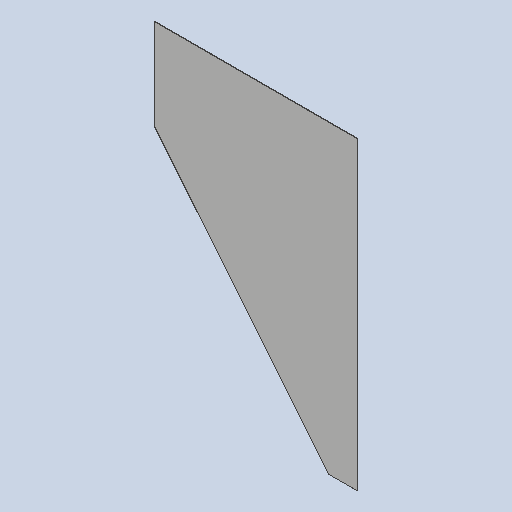
# Autodesk Inventor part: МОО 053 морда 3
Saved by Autodesk Inventor 2024.2 (Build 282272000, 272)
## iProperties
Created: 2024-06-08
Part Number: МОО 053 морда 3
Material: Generic
Document SubType Name: Sheet Metal
Designer: admin
Density: 1 g/cm^3
Sheet Metal Rule: Default
Appearance: Default
Author: admin
Autodesk Inventor part; units mm, degrees
ref_plane "YZ Plane" through (0, 0, 0) normal (1, 0, 0) x (0, 1, 0)
ref_plane "XZ Plane" through (0, 0, 0) normal (0, 1, 0) x (-1, 0, 0)
ref_plane "XY Plane" through (0, 0, 0) normal (0, 0, 1) x (1, 0, 0)
sketch "Sketch1" plane through (0, 0, 0) normal (0, 1, 0) x (-1, 0, 0)
  line L0 (0, 1200) -> (0, 0)
  line L1 (800, 843.901) -> (800, 1200)
  line L2 (800, 1200) -> (0, 1200)
  line L3 (800, 843.901) -> (113, 0)
  line L4 (113, 0) -> (0, 0)
  line L5 (685.2711, 713.7323) -> (114.1118, 12.1284)
  dimension "d0" = 1200
  dimension "d1" = 800
  dimension "d2" = 356.099
  dimension "d5" = 129.148
  dimension "d6" = 113
  measures "d0" distance of L0.end L0.start
  measures "d1" distance of L1.end L0.start
  measures "d2" distance of L1.start L1.end
  measures "d5" angle of L4 L3
  measures "d6" distance of L0.end L3.end
extrude "Plate1" add sketch "Sketch1" along normal blind 2
equation "\"d3\" = Thickness"
equation "\"BendRadius\" = Thickness"
equation "\"BendReliefWidth\" = Thickness"
equation "\"BendReliefDepth\" = 0.5 * Thickness"
equation "\"CornerReliefSize\" = 4 * Thickness"
equation "\"MinimumRemnant\" = 2 * Thickness"
equation "\"TransitionRadius\" = BendRadius"
equation "\"JacobiRadiusSize\" = BendRadius"
equation "\"GapSize\" = Thickness"
equation "\"Thickness\" = 2"
body "Solid1"
